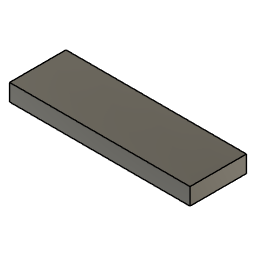
DiceHolder_Pin_V2 v2 (Autodesk Fusion 360 design; units mm, degrees)
Autodesk Fusion 360 part; units mm, degrees
sketch "Sketch1" plane through (0, 0, 0) normal (0, 0, 1) x (1, 0, 0)
  line L0 (-13, 2.5) -> (13, 2.5)
  line L1 (13, 2.5) -> (13, -2.5)
  line L2 (13, -2.5) -> (-13, -2.5)
  line L3 (-13, -2.5) -> (-13, 2.5)
  line L4 (-13, 2.5) -> (13, -2.5) construction
  line L5 (13, 2.5) -> (-13, -2.5) construction
  dimension "d1" = 26
  dimension "d2" = 5
  constraint horizontal L0
  constraint perpendicular L0 L1
  constraint parallel L0 L2
  constraint parallel L1 L3
  constraint coincident L4 origin
  constraint coincident L5 origin
  measures "d1" distance of L1.end L2.end
  measures "d2" distance of L0.end L1.end
extrude "Extrude1" add sketch "Sketch1" along normal blind 3
extrude "Extrude2" add 1 faces at (13, 0.8333, 1) along direction (1, 0, 0) blind 6
extrude "Extrude3" add 1 faces at (-2.3333, 2.5, 1) along direction (0, 1, 0) blind 5
